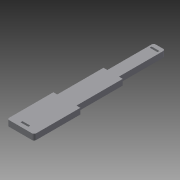
# Autodesk Inventor part: TENSOR
Saved by Autodesk Inventor 2015 (Build 190159000, 159)
## iProperties
Created: 2017-10-04
Part Number: TENSOR
Material: Generic
Document SubType Name: Modeling
Designer: Max
Density: 1 g/cm^3
Appearance: Default
Author: Max
Autodesk Inventor part; units mm, degrees
note: some values were not read from the file. Chosen so that the rebuilt part matches the saved one: sketch regions of "Extrusion1".
ref_plane "YZ Plane" through (0, 0, 0) normal (1, 0, 0) x (0, 1, 0)
ref_plane "XZ Plane" through (0, 0, 0) normal (0, 1, 0) x (-1, 0, 0)
ref_plane "XY Plane" through (0, 0, 0) normal (0, 0, 1) x (1, 0, 0)
sketch "Sketch1" plane through (0, 0, 0) normal (0, 0, 1) x (1, 0, 0)
  line L0 (0, 0) -> (-30, 0)
  line L1 (-30, 0) -> (-30, 360)
  line L2 (-30, 360) -> (0, 360)
  line L3 (0, 360) -> (0, 0)
  line L4 (-40, 240) -> (10, 240)
  line L5 (10, 240) -> (10, 0)
  line L6 (10, 0) -> (-40, 0)
  line L7 (-40, 0) -> (-40, 240)
  line L8 (-50, 120) -> (20, 120)
  line L9 (20, 120) -> (20, 0)
  line L10 (20, 0) -> (-50, 0)
  line L11 (-50, 0) -> (-50, 120)
  line L12 (-5, 10) -> (-25, 10)
  line L13 (-25, 10) -> (-25, 15)
  line L14 (-25, 15) -> (-5, 15)
  line L15 (-5, 15) -> (-5, 10)
  line L16 (-25, 350) -> (-5, 350)
  line L17 (-5, 350) -> (-5, 345)
  line L18 (-5, 345) -> (-25, 345)
  line L19 (-25, 345) -> (-25, 350)
  dimension "d0" = 30
  dimension "d1" = 360
  dimension "d2" = 50
  dimension "d3" = 70
  dimension "d4" = 20
  dimension "d5" = 5
  dimension "d6" = 5
  constraints: 40 end point, 10 parallel, 5 horizontal, 5 perpendicular, 1 point on line
  measures "d0" distance of L1.end L2.end
  measures "d1" distance of L0.end L1.end
  measures "d2" distance of L5.end L6.end
  measures "d3" distance of L9.end L10.end
  measures "d4" distance of L13.end L14.end
  measures "d5" distance of L12.end L13.end
  measures "d6" distance of L16.end L17.end
extrude "Extrusion1" add sketch "Sketch1" along normal blind 15
fillet "Fillet1" radius 5 4 edges at (-50, 0, 7.5) (20, 0, 7.5) (-30, 360, 7.5) (0, 360, 7.5)
body "Solid1"
